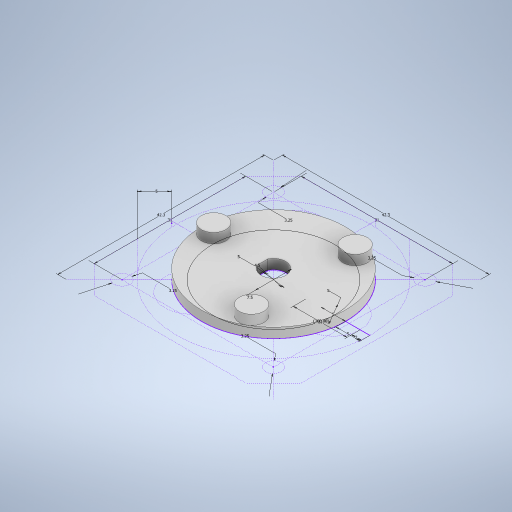
# Autodesk Inventor part: insert
Saved by Autodesk Inventor 2023 (Build 270158000, 158)
## iProperties
Created: 2022-12-06
Part Number: insert
Material: Generic
Document SubType Name: Modeling
Designer: Owner
Density: 1 g/cm^3
Appearance: Default
Author: Owner
Autodesk Inventor part; units mm, degrees
ref_plane "YZ Plane" through (0, 0, 0) normal (1, 0, 0) x (0, 1, 0)
ref_plane "XZ Plane" through (0, 0, 0) normal (0, 1, 0) x (-1, 0, 0)
ref_plane "XY Plane" through (0, 0, 0) normal (0, 0, 1) x (1, 0, 0)
sketch "Sketch1" plane through (0, 0, 0) normal (0, 1, 0) x (-1, 0, 0)
  line L0 (15.55, 0) -> (21.15, 0) construction
  line L1 (18.35, 0) -> (21.15, 0) construction
  arc A0 (2.25, 1.0897) -> (2.25, -1.0897) centre (0, 0) ccw construction
  circle A1 centre (0, 0) radius 2.25 construction
  line L2 (2.25, 0) -> (2.25, 1.0897) construction
  line L3 (2.25, 0) -> (2.25, -1.0897) construction
  line L4 (-15.5, 21.15) -> (15.5, 21.15) construction
  line L5 (21.15, 15.5) -> (21.15, -15.5) construction
  line L6 (15.5, -21.15) -> (-15.5, -21.15) construction
  line L7 (-21.15, -15.5) -> (-21.15, 15.5) construction
  line L8 (-21.15, 21.15) -> (21.15, -21.15) construction
  line L9 (21.15, 21.15) -> (-21.15, -21.15) construction
  line L10 (-15.5, 15.5) -> (15.5, 15.5) construction
  line L11 (15.5, 15.5) -> (15.5, -15.5) construction
  line L12 (15.5, -15.5) -> (-15.5, -15.5) construction
  line L13 (-15.5, -15.5) -> (-15.5, 15.5) construction
  line L14 (-15.5, 15.5) -> (15.5, -15.5) construction
  line L15 (15.5, 15.5) -> (-15.5, -15.5) construction
  circle A2 centre (15.5, 15.5) radius 1.625 construction
  circle A3 centre (15.5, -15.5) radius 1.625 construction
  circle A4 centre (-15.5, -15.5) radius 1.625 construction
  circle A5 centre (-15.5, 15.5) radius 1.625 construction
  line L16 (15.5, -15.5) -> (15.5, -21.15) construction
  line L17 (21.15, -15.5) -> (15.5, -21.15) construction
  line L18 (-15.5, -21.15) -> (-21.15, -15.5) construction
  line L19 (-21.15, 15.5) -> (-15.5, 21.15) construction
  line L20 (15.5, 21.15) -> (21.15, 15.5) construction
  line L21 (0, -15.5) -> (0, -21.15) construction
  line L22 (0, -15.5) -> (0, -18.325) construction
  line L23 (0, -18.325) -> (0, -21.15) construction
  circle A6 centre (0, 0) radius 19.7375 construction
  line L24 (-15.5, -21.15) -> (15.5, -21.15) construction
  line L25 (-13.9565, -13.9565) -> (-6.763, -21.15) construction
  line L26 (0, 0) -> (7.7782, -7.7782) construction
  line L27 (13.9565, 13.9565) -> (21.15, 6.763) construction
  line L28 (-1.1373, -19.7047) -> (0.308, -21.15) construction
  line L29 (19.7047, 1.1373) -> (21.15, -0.308) construction
  arc A7 (2.25, 1.0897) -> (2.25, -1.0897) centre (0, 0) ccw
  line L30 (2.25, 1.0897) -> (2.25, -1.0897)
  circle A8 centre (0, 0) radius 3.75
  line L31 (-19.7375, 0) -> (-17.7375, 0)
  line L32 (-19.7375, 0) -> (-14.7375, 0)
  line L33 (-17.7375, 0) -> (-6.7375, 0)
  circle A9 centre (-12.2375, 0) radius 5.5 construction
  circle A10 centre (-12.2375, 0) radius 2.5
  line L34 (-12.2375, 2.5) -> (-1.8548, 2.5) construction
  line L35 (-12.2375, -2.5) -> (-1.8548, -2.5) construction
  line L36 (3.9537, -11.848) -> (-1.2377, -2.8563) construction
  circle A11 centre (6.1187, -10.598) radius 2.5
  line L37 (8.2838, -9.348) -> (3.0924, -0.3563) construction
  circle A12 centre (6.1187, -10.598) radius 5.5 construction
  line L38 (8.2838, 9.348) -> (3.0924, 0.3563) construction
  circle A13 centre (6.1188, 10.598) radius 2.5
  line L39 (3.9537, 11.848) -> (-1.2377, 2.8563) construction
  circle A14 centre (6.1188, 10.598) radius 5.5 construction
  circle A15 centre (0, 0) radius 14.7375
  circle A16 centre (0, 0) radius 9.7375
  point P0 (-10.421, -10.421)
  point P1 (10.421, 10.421)
  point P2 (20.4274, 0.4146)
  point P3 (15.5, 12.2196)
  point P4 (15.5, 12.413)
  point P5 (-12.413, -15.5)
  point P6 (-12.2196, -15.5)
  point P7 (0, -20.842)
  point P8 (21.15, -0.308)
  point P9 (3.3687, -5.8348)
  point P10 (3.3688, 5.8348)
  dimension "d9" = 4.5
  dimension "d8" = 5
  dimension "d10" = 42.3
  dimension "d11" = 42.3
  dimension "d12" = 31
  dimension "d13" = 31
  dimension "d15" = 3.25
  dimension "d16" = 3.25
  dimension "d17" = 3.25
  dimension "d18" = 3.25
  dimension "d20" = 5
  dimension "d21" = 7.5
  dimension "d22" = 2
  dimension "d23" = 5
  dimension "d24" = 11
  dimension "d25" = 5
  dimension "d28" = 360
  dimension "d31" = 5
  constraints: 80 end point, 14 point on circle, 12 centre point, 11 coincident, 10 midpoint, 10 point on line, 7 perpendicular, 6 horizontal, 4 parallel, 4 symmetric about line, 3 collinear, 3 horizontal alignment, 2 tangent, 2 vertical, 1 concentric, 46 other
  measures "d8" diameter of A0
  measures "d10" distance of L8.end L9.end
  measures "d11" distance of L9.start L8.end
  measures "d12" distance of L11.end L12.end
  measures "d13" distance of L10.end L11.end
  measures "d15" diameter of A2
  measures "d16" diameter of A3
  measures "d17" diameter of A4
  measures "d18" diameter of A5
  measures "d20" distance from line of point (20.427, 0.415) L27
  measures "d21" diameter of A8
  measures "d22" distance of L31.start L31.end
  measures "d23" distance of L31.start L32.end
  measures "d24" distance of L31.end L33.end
  measures "d25" diameter of A10
extrude "Extrusion1" add sketch "Sketch1" along normal blind 2 contours A8 | A10 L33 | A15 A13 A16 A10 | L33 A10 | A10 A16 A11 A15 | A16 | A15 A11 A16 A13 | A13 | A11
sketch "Sketch2" plane through (0, 2, 0) normal (0, 1, 0) x (1, 0, 0)
  line L0 (15.55, 0) -> (21.15, 0) construction
  line L1 (18.35, 0) -> (21.15, 0) construction
  arc A0 (2.25, 1.0897) -> (2.25, -1.0897) centre (0, 0) ccw construction
  circle A1 centre (0, 0) radius 2.25 construction
  line L2 (2.25, 0) -> (2.25, 1.0897) construction
  line L3 (2.25, 0) -> (2.25, -1.0897) construction
  line L4 (-15.5, 21.15) -> (15.5, 21.15) construction
  line L5 (21.15, 15.5) -> (21.15, -15.5) construction
  line L6 (15.5, -21.15) -> (-15.5, -21.15) construction
  line L7 (-21.15, -15.5) -> (-21.15, 15.5) construction
  line L8 (-21.15, 21.15) -> (21.15, -21.15) construction
  line L9 (21.15, 21.15) -> (-21.15, -21.15) construction
  line L10 (-15.5, 15.5) -> (15.5, 15.5) construction
  line L11 (15.5, 15.5) -> (15.5, -15.5) construction
  line L12 (15.5, -15.5) -> (-15.5, -15.5) construction
  line L13 (-15.5, -15.5) -> (-15.5, 15.5) construction
  line L14 (-15.5, 15.5) -> (15.5, -15.5) construction
  line L15 (15.5, 15.5) -> (-15.5, -15.5) construction
  circle A2 centre (15.5, 15.5) radius 1.625 construction
  circle A3 centre (15.5, -15.5) radius 1.625 construction
  circle A4 centre (-15.5, -15.5) radius 1.625 construction
  circle A5 centre (-15.5, 15.5) radius 1.625 construction
  line L16 (15.5, -15.5) -> (15.5, -21.15) construction
  line L17 (21.15, -15.5) -> (15.5, -21.15) construction
  line L18 (-15.5, -21.15) -> (-21.15, -15.5) construction
  line L19 (-21.15, 15.5) -> (-15.5, 21.15) construction
  line L20 (15.5, 21.15) -> (21.15, 15.5) construction
  line L21 (0, -15.5) -> (0, -21.15) construction
  line L22 (0, -15.5) -> (0, -18.325) construction
  line L23 (0, -18.325) -> (0, -21.15) construction
  circle A6 centre (0, 0) radius 19.7375 construction
  line L24 (-15.5, -21.15) -> (15.5, -21.15) construction
  line L25 (-13.9565, -13.9565) -> (-6.763, -21.15) construction
  line L26 (0, 0) -> (7.7782, -7.7782) construction
  line L27 (13.9565, 13.9565) -> (21.15, 6.763) construction
  line L28 (-1.1373, -19.7047) -> (0.308, -21.15) construction
  line L29 (19.7047, 1.1373) -> (21.15, -0.308) construction
  arc A7 (2.25, 1.0897) -> (2.25, -1.0897) centre (0, 0) ccw
  line L30 (2.25, 1.0897) -> (2.25, -1.0897)
  circle A8 centre (0, 0) radius 3.75
  line L31 (-19.7375, 0) -> (-17.7375, 0)
  line L32 (-19.7375, 0) -> (-14.7375, 0)
  line L33 (-17.7375, 0) -> (-6.7375, 0)
  circle A9 centre (-12.2375, 0) radius 5.5 construction
  circle A10 centre (-12.2375, 0) radius 2.5
  line L34 (-12.2375, 2.5) -> (-1.8548, 2.5) construction
  line L35 (-12.2375, -2.5) -> (-1.8548, -2.5) construction
  line L36 (3.9537, -11.848) -> (-1.2377, -2.8563) construction
  circle A11 centre (6.1187, -10.598) radius 2.5
  line L37 (8.2838, -9.348) -> (3.0924, -0.3563) construction
  circle A12 centre (6.1187, -10.598) radius 5.5 construction
  line L38 (8.2838, 9.348) -> (3.0924, 0.3563) construction
  circle A13 centre (6.1188, 10.598) radius 2.5
  line L39 (3.9537, 11.848) -> (-1.2377, 2.8563) construction
  circle A14 centre (6.1188, 10.598) radius 5.5 construction
  circle A15 centre (0, 0) radius 14.7375
  circle A16 centre (0, 0) radius 9.7375
  point P0 (-10.421, -10.421)
  point P1 (20.4274, 0.4146)
  point P2 (10.421, 10.421)
  point P3 (15.5, 12.2196)
  point P4 (15.5, 12.413)
  point P5 (-12.413, -15.5)
  point P6 (-12.2196, -15.5)
  point P7 (0, -20.842)
  point P8 (21.15, -0.308)
  point P9 (3.3687, -5.8348)
  point P10 (3.3688, 5.8348)
  dimension "d37" = 4.5
  dimension "d36" = 5
  dimension "d38" = 42.3
  dimension "d39" = 42.3
  dimension "d40" = 31
  dimension "d41" = 31
  dimension "d42" = 3.25
  dimension "d43" = 3.25
  dimension "d44" = 3.25
  dimension "d45" = 3.25
  dimension "d46" = 5
  dimension "d47" = 7.5
  dimension "d48" = 2
  dimension "d49" = 5
  dimension "d50" = 11
  dimension "d51" = 5
  dimension "d52" = 360
  dimension "d53" = 5
  constraints: 80 end point, 14 point on circle, 12 centre point, 11 coincident, 10 midpoint, 10 point on line, 7 perpendicular, 6 horizontal, 4 parallel, 4 symmetric about line, 3 collinear, 3 horizontal alignment, 2 tangent, 2 vertical, 1 concentric, 46 other
  measures "d36" diameter of A0
  measures "d38" distance of L8.end L9.end
  measures "d39" distance of L9.start L8.end
  measures "d40" distance of L11.end L12.end
  measures "d41" distance of L10.end L11.end
  measures "d42" diameter of A2
  measures "d43" diameter of A3
  measures "d44" diameter of A4
  measures "d45" diameter of A5
  measures "d46" distance from line of point (20.427, 0.415) L27
  measures "d47" diameter of A8
  measures "d48" distance of L31.start L31.end
  measures "d49" distance of L31.start L32.end
  measures "d50" distance of L31.end L33.end
  measures "d51" diameter of A10
extrude "Extrusion2" add sketch "Sketch2" along normal blind 2 contours A10 L33 | L33 A10 | A13 | A11
body "Solid1"
